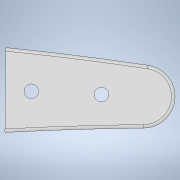
# Autodesk Inventor part: LegEnd_Right_Head
Saved by Autodesk Inventor 2020.3 (Build 243373000, 373)
## iProperties
Created: 2021-02-18
Part Number: LegEnd_Right_Head
Material: Generic
Document SubType Name: Modeling
Designer: sanyi
Density: 1 g/cm^3
Appearance: Default
Author: sanyi
Autodesk Inventor part; units mm, degrees
ref_plane "YZ Plane" through (0, 0, 0) normal (1, 0, 0) x (0, 1, 0)
ref_plane "XZ Plane" through (0, 0, 0) normal (0, 1, 0) x (-1, 0, 0)
ref_plane "XY Plane" through (0, 0, 0) normal (0, 0, 1) x (1, 0, 0)
sketch "Sketch1" plane through (0, 0, 0) normal (0, 1, 0) x (-1, 0, 0)
  line L0 (0, 0) -> (-4, 0)
  line L1 (0, 0) -> (0, 36.6)
  line L2 (-24.4, 0) -> (-24.4, 6) construction
  line L3 (-18.4, 6) -> (-6, 6)
  line L4 (-6, 6) -> (-6, 30.6)
  line L5 (-6, 30.6) -> (-18.4, 30.6)
  line L6 (-18.4, 30.6) -> (-18.4, 6)
  line L7 (-24.4, 36.6) -> (-23.6295, 36.6) construction
  arc A0 (-20.163, 113.1038) -> (-23.4834, 116.9404) centre (-20, 116.6) ccw construction
  line L8 (-12.2, 4.1) -> (-12.2, 32.5) construction
  line L9 (-26.8761, 4.1) -> (8.0494, 4.1) construction
  line L10 (-27.3708, 32.5) -> (4.7796, 32.5) construction
  line L11 (-27.5308, 18.3) -> (1.4723, 18.3) construction
  arc A1 (-16.5002, 116.6381) -> (-9, 36.6) centre (470.9644, 121.9469) ccw construction
  line L12 (-23.6295, 36.6) -> (-13.0622, 36.6)
  line L13 (-9, 36.6) -> (0, 36.6)
  line L14 (-21.9951, 96.4905) -> (-19.8751, 96.6)
  line L15 (-19.8751, 96.6) -> (-15.8804, 96.8063) construction
  line L16 (-21.9951, 96.4905) -> (-25.9754, 96.8873) construction
  line L17 (-13.0622, 36.6) -> (-9.123, 37.2946) construction
  line L18 (-20, 116.6) -> (-16.5, 116.6) construction
  line L19 (-20, 116.6) -> (-20.7452, 100.6174) construction
  line L20 (-18.4, 6) -> (-24.4, 6)
  line L21 (-6, 6) -> (0, 6)
  arc A2 (-17.4, 0) -> (-14.7466, -6.9504) centre (-6.9703, 0) ccw
  arc A3 (-9.6573, 0) -> (-14.7466, -6.9504) centre (-0.5472, -12.0091) ccw
  arc A4 (-20.4, 0) -> (-13, -12) centre (-6.9703, 0) ccw
  arc A5 (-4, 0) -> (-13, -12) centre (1.9602, -13.8452) ccw
  line L22 (-14.7466, -6.9504) -> (-16.9833, -8.9496) construction
  line L23 (-14.7466, -6.9504) -> (-11.9734, -8.0949) construction
  line L24 (-20.4, 0) -> (-24.4, 0)
  line L25 (-17.4, 0) -> (-20.4, 0) construction
  line L26 (-9.6573, 0) -> (-17.4, 0)
  line L27 (-7.7289, -2.2981) -> (-9.6573, 0) construction
  arc A6 (-23.4834, 116.9404) -> (-20.163, 113.1038) centre (-20, 116.6) ccw construction
  line L28 (-21.4, -3.4679) -> (-21.4, 37.7463) construction
  line L29 (-24.4, 19.6) -> (-18.4, 19.6)
  line L30 (-6, 19.6) -> (0, 19.6)
  line L31 (-29.0378, 12.8) -> (2.5913, 12.8) construction
  arc A7 (-23.4618, 117.1157) -> (-24.4, 0) centre (391.9533, 55.2262) ccw construction
  arc A8 (-21.9951, 96.4905) -> (-23.6295, 36.6) centre (391.9533, 55.2262) ccw
  arc A9 (-19.8751, 96.6) -> (-13.0622, 36.6) centre (470.9644, 121.9469) ccw
  line L32 (-20.7452, 100.6174) -> (-20.9351, 96.5453) construction
  line L33 (-24.4, 6) -> (-24.4, 19.6)
  line L34 (-24.4, 19.6) -> (-24.4, 36.6) construction
  arc A10 (-15.5003, 116.649) -> (-8.1614, 37.6) centre (470.9644, 121.9469) ccw
  line L35 (-8.1614, 37.6) -> (1, 37.6)
  line L36 (1, 37.6) -> (1, -1)
  line L37 (1, -1) -> (-3.7902, -1)
  arc A11 (-3.7902, -1) -> (-12.1087, -13.4838) centre (1.9602, -13.8452) ccw
  arc A12 (-21.3653, -1) -> (-12.1087, -13.4838) centre (-6.9703, 0) ccw
  line L38 (-21.3653, -1) -> (-25.2752, -1)
  arc A13 (-24.4509, 117.2631) -> (-25.2752, -1) centre (391.9533, 55.2262) ccw
  arc A14 (-15.5003, 116.649) -> (-24.4509, 117.2631) centre (-20, 116.6) ccw
  line L39 (-15.8804, 96.8063) -> (-14.8817, 96.8579)
  line L40 (-25.9754, 96.8873) -> (-26.9704, 96.9865)
  line L41 (-26.9704, 96.9865) -> (-14.8817, 96.8579)
  point P0 (-20.2795, 110.6065)
  dimension "d4" = 6
  dimension "d5" = 24.6
  dimension "d6" = 12.4
  dimension "d7" = 6
  dimension "d15" = 7
  dimension "d17" = 9
  dimension "d21" = 20
  dimension "d23" = 80
  dimension "d24" = 20
  dimension "d29" = 170
  dimension "d30" = 6
  dimension "d31" = 10
  dimension "d43" = 4
  dimension "d44" = 3
  dimension "d45" = 4
  dimension "d50" = 13
  dimension "d51" = 12
  dimension "d52" = 130
  dimension "d89" = 6.8
  dimension "d90" = 28.4
  dimension "d107" = 420
  dimension "d108" = 4
  dimension "d109" = 4
  dimension "d114" = 1
  dimension "d115" = 1
  constraints: 85 end point, 43 point on circle, 15 centre point, 14 point on line, 9 horizontal, 9 line through centre, 9 perpendicular, 6 vertical, 5 collinear, 3 equal length, 3 parallel, 2 tangent, 1 concentric, 1 equal radius, 1 midpoint, 15 other
  measures "d4" distance between parallel lines of L0 L3
  measures "d5" distance between parallel lines of L5 L3
  measures "d6" distance between parallel lines of L4 L6
  measures "d7" distance between parallel lines of L1 L4
  measures "d15" diameter of A0
  measures "d17" distance of L1.end L13.start
  measures "d21" vertical distance of L18.start L14.end
  measures "d23" vertical distance of L18.start L1.end
  measures "d24" horizontal distance of L1.end L18.start
  measures "d29" angle of L12 L17
  measures "d30" distance of L18.start point (-20.279, 110.607)
  measures "d31" distance of L19.end point (-20.279, 110.607)
  measures "d43" distance of L2.start L24.start
  measures "d44" distance of L25.start L24.start
  measures "d45" distance of L0.start L0.end
  measures "d50" distance from line of L1 A4.end
  measures "d51" distance from line of L24 A4.end
  measures "d52" angle of L26 L27
  measures "d89" distance between parallel lines of L3 L31
  measures "d90" distance between parallel lines of L9 L10
  measures "d107" radius of A7
  measures "d108" radial gap between concentric circles of A7 A8
  measures "d109" distance of L12.end L17.end
  measures "d114" radial gap between concentric circles of A1 A10
  measures "d115" radial gap between concentric circles of A0 A14
extrude "Extrusion4" add sketch "Sketch1" along normal blind 8 contours A10 L41 A13 A14
shell "Shell1" thickness 1 removed faces 1 at (22.9409, 5.3333, 96.9436)
hole "Hole6" at (12.2, 0, 4.1) at (12.2, 0, 32.5) at (20.2795, 0, 110.6065) at (20.7452, 0, 100.6174) direction (0, 1, 0) diameter 2.1 end through all
fillet "Fillet12" radius 0.5 6 edges at (19.692, 8, 121.0894) (15.2917, 8, 106.7503) (25.8337, 8, 107.1401) (19.692, 0, 121.0894) (15.2917, 0, 106.7503) (25.8337, 0, 107.1401)
body "Solid2"
